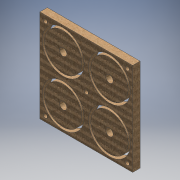
# Autodesk Inventor part: MotorSiliconeMold_2
Saved by Autodesk Inventor 2016 (Build 200138000, 138)
## iProperties
Created: 2015-12-06
Part Number: MotorSiliconeMold_2
Material: MDF Medium Density Fiberboard
Document SubType Name: Modeling
Designer: DonMo
Density: 0.8 g/cm^3
Appearance: Cardboard - Corrugated
BearingDiameter: 24.000 mm
WoodThickness: 6.390 mm
BearingWidth: 7.000 mm
BearingShaftDiameter: 8.000 mm
ZipTieWidth: 2.500 mm
ZipTieThickness: 1.100 mm
ZipTieClearance: 1.000 mm
ZipTieDistance: 10.000 mm
BearingHolderHeight: 13.100 mm
MotorWidth: 37.000 mm
SupportClearance: 5.000 mm
MotorShaftWidth: 12.000 mm
CouplingWidth: 0.375 in
CouplingDiameter: 0.870 in
DiskGap: 75.835 mm
d28: 360.00 deg
SiliconeRingDiameter: 36.224 mm
DowlDiameter: 6.300 mm
HoldScrewDiameter: 3.430 mm
VccumCoverSize: 80.000 mm
SiliconeOverlapThickness: 2.000 mm
Author: DonMo
Autodesk Inventor part; units mm, degrees
ref_plane "YZ Plane" through (0, 0, 0) normal (1, 0, 0) x (0, 1, 0)
ref_plane "XZ Plane" through (0, 0, 0) normal (0, 1, 0) x (-1, 0, 0)
ref_plane "XY Plane" through (0, 0, 0) normal (0, 0, 1) x (1, 0, 0)
sketch "Sketch1" plane through (0, 0, 0) normal (0, 1, 0) x (-1, 0, 0)
  line L0 (0, 0) -> (-80, 0)
  line L1 (-80, 0) -> (-80, 80)
  line L2 (-80, 80) -> (0, 80)
  line L3 (0, 80) -> (0, 0)
  line L4 (0, 40) -> (-40, 40) construction
  line L5 (-40, 40) -> (-40, 80) construction
  line L6 (-40, 40) -> (-80, 40) construction
  line L7 (-40, 40) -> (-40, 0) construction
  circle A0 centre (-20, 20) radius 18.1118
  circle A1 centre (-20, 20) radius 16.1118
  circle A2 centre (-20, 20) radius 3.15
  circle A3 centre (-4.6447, 4.6447) radius 1.715
  line L8 (-40, 40) -> (0, 0) construction
  circle A4 centre (-20, 60) radius 18.1118
  circle A5 centre (-20, 60) radius 16.1118
  circle A6 centre (-20, 60) radius 3.15
  circle A7 centre (-4.6447, 75.3553) radius 1.715
  circle A8 centre (-60, 20) radius 18.1118
  circle A9 centre (-60, 20) radius 16.1118
  circle A10 centre (-60, 20) radius 3.15
  circle A11 centre (-75.3553, 4.6447) radius 1.715
  circle A12 centre (-75.3553, 75.3553) radius 1.715
  circle A13 centre (-60, 60) radius 18.1118
  circle A14 centre (-60, 60) radius 16.1118
  circle A15 centre (-60, 60) radius 3.15
  circle A16 centre (-40, 40) radius 1.715
  point P0 (-20, 40)
  point P1 (-40, 20)
  dimension "d0" = 80
  dimension "d1" = 80
  dimension "d2" = 36.2235
  dimension "d3" = 2
  dimension "d4" = 6.3
  dimension "d5" = 3.43
  dimension "d6" = 50
  dimension "d7" = 3.43
  constraints: 18 end point, 17 centre point, 12 symmetric about line, 9 coincident, 6 midpoint, 3 parallel, 2 horizontal, 1 horizontal alignment, 1 perpendicular, 1 point on line, 1 vertical alignment, 12 other
  measures "d0" distance of L1.end L2.end
  measures "d1" distance of L0.end L1.end
  measures "d2" diameter of A0
  measures "d3" radial gap between concentric circles of A0 A1
  measures "d4" diameter of A2
  measures "d5" diameter of A3
  measures "d6" distance of L4.end A3.centre
  measures "d7" diameter of A16
extrude "Extrusion1" add sketch "Sketch1" along normal blind 6.39
equation "\"d0\" = VccumCoverSize"
equation "\"d1\" = VccumCoverSize"
equation "\"d2\" = SiliconeRingDiameter"
equation "\"d3\" = SiliconeOverlapThickness"
equation "\"d4\" = DowlDiameter"
equation "\"d5\" = HoldScrewDiameter"
equation "\"d7\" = HoldScrewDiameter"
equation "\"d8\" = WoodThickness"
equation "\"SiliconeOverlapThickness\" = 2"
equation "\"VccumCoverSize\" = 80"
equation "\"SiliconeRingDiameter\" = 36.2235"
equation "\"DowlDiameter\" = 6.3"
equation "\"HoldScrewDiameter\" = 3.43"
equation "\"WoodThickness\" = 6.39"
body "Solid1"
